Autodesk Inventor part; units mm, degrees
(part 4 of 4)
extrude "Extrusion2" cut sketch "Sketch2" against normal blind 1.5875 contours A0 L8 A2 L7 A1 L6 | L9 A4 L10 A5 L11 A3 | L12 A7 L14 A6 L13 A8 | L15 A11 L17 A10 L16 A9 | L18 A13 L20 A12 L19 A14 | L21 A17 L23 A16 L22 A15 | L24 A19 L26 A18 L25 A20 | L27 A23 L29 A22 L28 A21 | L30 A25 L32 A24 L31 A26 | L33 A29 L35 A28 L34 A27 | L36 A31 L38 A30 L37 A32 | L39 A35 L41 A34 L40 A33 | L42 A37 L44 A36 L43 A38 | L45 A41 L47 A40 L46 A39 | L48 A43 L50 A42 L49 A44 | L51 A47 L53 A46 L52 A45 | L54 A49 L56 A48 L55 A50 | L57 A53 L59 A52 L58 A51 | L60 A55 L62 A54 L61 A56 | L63 A59 L65 A58 L64 A57 | L66 A61 L68 A60 L67 A62 | L69 A65 L71 A64 L70 A63 | L72 A67 L74 A66 L73 A68 | L75 A71 L77 A70 L76 A69 | L78 A73 L80 A72 L79 A74 | L81 A77 L83 A76 L82 A75 | L84 A79 L86 A78 L85 A80 | L87 A83 L89 A82 L88 A81 | L90 A85 L92 A84 L91 A86 | L93 A89 L95 A88 L94 A87 | L96 A91 L98 A90 L97 A92 | L99 A95 L101 A94 L100 A93 | L102 A97 L104 A96 L103 A98 | L105 A101 L107 A100 L106 A99 | L108 A103 L110 A102 L109 A104 | L111 A107 L113 A106 L112 A105 | L114 A109 L116 A108 L115 A110 | L117 A113 L119 A112 L118 A111 | L120 A115 L122 A114 L121 A116 | L123 A119 L125 A118 L124 A117 | L126 A121 L128 A120 L127 A122 | L129 A125 L131 A124 L130 A123 | L132 A127 L134 A126 L133 A128 | L135 A131 L137 A130 L136 A129 | L138 A133 L140 A132 L139 A134 | L141 A137 L143 A136 L142 A135 | L144 A139 L146 A138 L145 A140 | L147 A143 L149 A142 L148 A141 | L150 A145 L152 A144 L151 A146 | L153 A149 L155 A148 L154 A147 | L156 A151 L158 A150 L157 A152 | L159 A155 L161 A154 L160 A153 | L162 A157 L164 A156 L163 A158 | L165 A161 L167 A160 L166 A159 | L168 A163 L170 A162 L169 A164 | L171 A167 L173 A166 L172 A165 | L174 A169 L176 A168 L175 A170 | L177 A173 L179 A172 L178 A171 | L180 A175 L182 A174 L181 A176 | L183 A179 L185 A178 L184 A177 | L186 A181 L188 A180 L187 A182 | L189 A185 L191 A184 L190 A183 | L192 A187 L194 A186 L193 A188 | L195 A191 L197 A190 L196 A189 | L198 A193 L200 A192 L199 A194 | L201 A197 L203 A196 L202 A195 | L204 A199 L206 A198 L205 A200 | L207 A203 L209 A202 L208 A201 | L210 A205 L212 A204 L211 A206 | L213 A209 L215 A208 L214 A207 | L216 A211 L218 A210 L217 A212 | L219 A215 L221 A214 L220 A213 | L222 A217 L224 A216 L223 A218 | L225 A221 L227 A220 L226 A219 | L228 A223 L230 A222 L229 A224 | L231 A227 L233 A226 L232 A225 | L234 A229 L236 A228 L235 A230 | L237 A233 L239 A232 L238 A231 | L240 A235 L242 A234 L241 A236 | L243 A239 L245 A238 L244 A237 | L246 A241 L248 A240 L247 A242 | L249 A245 L251 A244 L250 A243 | L252 A247 L254 A246 L253 A248 | L255 A251 L257 A250 L256 A249 | L258 A253 L260 A252 L259 A254 | L261 A257 L263 A256 L262 A255 | L264 A259 L266 A258 L265 A260 | L267 A263 L269 A262 L268 A261 | L270 A265 L272 A264 L271 A266 | L273 A269 L275 A268 L274 A267 | L276 A271 L278 A270 L277 A272 | L279 A275 L281 A274 L280 A273 | L282 A277 L284 A276 L283 A278 | L285 A281 L287 A280 L286 A279 | L288 A283 L290 A282 L289 A284 | L291 A287 L293 A286 L292 A285 | L294 A289 L296 A288 L295 A290 | L297 A293 L299 A292 L298 A291 | L300 A295 L302 A294 L301 A296 | L303 A299 L305 A298 L304 A297 | L306 A301 L308 A300 L307 A302 | L309 A305 L311 A304 L310 A303 | L312 A307 L314 A306 L313 A308 | L315 A311 L317 A310 L316 A309 | L318 A313 L320 A312 L319 A314 | L321 A317 L323 A316 L322 A315 | L324 A319 L326 A318 L325 A320 | L327 A323 L329 A322 L328 A321 | L330 A325 L332 A324 L331 A326 | L333 A329 L335 A328 L334 A327 | L336 A331 L338 A330 L337 A332 | L339 A335 L341 A334 L340 A333 | L342 A337 L344 A336 L343 A338 | L345 A341 L347 A340 L346 A339 | L348 A343 L350 A342 L349 A344 | L351 A347 L353 A346 L352 A345 | L354 A349 L356 A348 L355 A350 | L357 A353 L359 A352 L358 A351 | L360 A355 L362 A354 L361 A356 | L363 A359 L365 A358 L364 A357 | L366 A361 L368 A360 L367 A362 | L369 A365 L371 A364 L370 A363 | L372 A367 L374 A366 L373 A368 | L375 A371 L377 A370 L376 A369 | L378 A373 L380 A372 L379 A374 | L381 A377 L383 A376 L382 A375 | L384 A379 L386 A378 L385 A380 | L387 A383 L389 A382 L388 A381 | L390 A385 L392 A384 L391 A386 | L393 A389 L395 A388 L394 A387 | L396 A391 L398 A390 L397 A392 | L399 A395 L401 A394 L400 A393 | L402 A397 L404 A396 L403 A398 | L405 A401 L407 A400 L406 A399 | L408 A403 L410 A402 L409 A404 | L411 A407 L413 A406 L412 A405 | L414 A409 L416 A408 L415 A410 | L417 A413 L419 A412 L418 A411 | L420 A415 L422 A414 L421 A416 | L423 A419 L425 A418 L424 A417 | L426 A421 L428 A420 L427 A422 | L429 A425 L431 A424 L430 A423 | L432 A427 L434 A426 L433 A428 | L435 A431 L437 A430 L436 A429 | L438 A433 L440 A432 L439 A434 | L441 A437 L443 A436 L442 A435 | L444 A439 L446 A438 L445 A440 | L447 A443 L449 A442 L448 A441 | L450 A445 L452 A444 L451 A446 | L453 A449 L455 A448 L454 A447 | L456 A451 L458 A450 L457 A452 | L459 A455 L461 A454 L460 A453 | L462 A457 L464 A456 L463 A458 | L465 A461 L467 A460 L466 A459 | L468 A463 L470 A462 L469 A464 | L471 A467 L473 A466 L472 A465 | L474 A469 L476 A468 L475 A470 | L477 A473 L479 A472 L478 A471 | L480 A475 L482 A474 L481 A476 | L483 A479 L485 A478 L484 A477 | L486 A481 L488 A480 L487 A482 | L489 A485 L491 A484 L490 A483 | L492 A487 L494 A486 L493 A488 | L495 A491 L497 A490 L496 A489 | L498 A493 L500 A492 L499 A494 | L501 A497 L503 A496 L502 A495 | L504 A499 L506 A498 L505 A500 | L507 A503 L509 A502 L508 A501 | L510 A505 L512 A504 L511 A506 | L513 A509 L515 A508 L514 A507 | L516 A511 L518 A510 L517 A512 | L519 A515 L521 A514 L520 A513 | L522 A517 L524 A516 L523 A518 | L525 A521 L527 A520 L526 A519 | L528 A523 L530 A522 L529 A524 | L531 A527 L533 A526 L532 A525 | L534 A529 L536 A528 L535 A530 | L537 A533 L539 A532 L538 A531 | L540 A535 L542 A534 L541 A536 | L543 A539 L545 A538 L544 A537 | L546 A541 L548 A540 L547 A542 | L549 A545 L551 A544 L550 A543 | L552 A547 L554 A546 L553 A548 | L555 A551 L557 A550 L556 A549 | L558 A553 L560 A552 L559 A554 | L561 A557 L563 A556 L562 A555 | L564 A559 L566 A558 L565 A560 | L567 A563 L569 A562 L568 A561 | L570 A565 L572 A564 L571 A566 | L573 A569 L575 A568 L574 A567 | L576 A571 L578 A570 L577 A572 | L579 A575 L581 A574 L580 A573 | L582 A577 L584 A576 L583 A578 | L585 A581 L587 A580 L586 A579 | L588 A583 L590 A582 L589 A584 | L591 A587 L593 A586 L592 A585 | L594 A589 L596 A588 L595 A590 | L597 A593 L599 A592 L598 A591 | L600 A595 L602 A594 L601 A596 | L603 A599 L605 A598 L604 A597 | L606 A601 L608 A600 L607 A602 | L609 A605 L611 A604 L610 A603 | L612 A607 L614 A606 L613 A608 | L615 A611 L617 A610 L616 A609 | L618 A613 L620 A612 L619 A614 | L621 A617 L623 A616 L622 A615 | L624 A619 L626 A618 L625 A620 | L627 A623 L629 A622 L628 A621 | L630 A625 L632 A624 L631 A626 | L633 A629 L635 A628 L634 A627 | L636 A631 L638 A630 L637 A632 | L639 A635 L641 A634 L640 A633 | L642 A637 L644 A636 L643 A638 | L645 A641 L647 A640 L646 A639 | L648 A643 L650 A642 L649 A644 | L651 A647 L653 A646 L652 A645 | L654 A649 L656 A648 L655 A650 | L657 A653 L659 A652 L658 A651 | L660 A655 L662 A654 L661 A656 | L663 A659 L665 A658 L664 A657 | L666 A661 L668 A660 L667 A662 | L669 A665 L671 A664 L670 A663 | L672 A667 L674 A666 L673 A668 | L675 A671 L677 A670 L676 A669 | L678 A673 L680 A672 L679 A674 | L681 A677 L683 A676 L682 A675 | L684 A679 L686 A678 L685 A680 | L687 A683 L689 A682 L688 A681 | L690 A685 L692 A684 L691 A686 | L693 A689 L695 A688 L694 A687 | L696 A691 L698 A690 L697 A692 | L699 A695 L701 A694 L700 A693 | L702 A697 L704 A696 L703 A698 | L705 A701 L707 A700 L706 A699 | L708 A703 L710 A702 L709 A704 | L711 A707 L713 A706 L712 A705 | L714 A709 L716 A708 L715 A710 | L717 A713 L719 A712 L718 A711 | L720 A715 L722 A714 L721 A716 | L723 A719 L725 A718 L724 A717 | L726 A721 L728 A720 L727 A722 | L729 A725 L731 A724 L730 A723 | L732 A727 L734 A726 L733 A728 | L735 A731 L737 A730 L736 A729 | L738 A733 L740 A732 L739 A734 | L741 A737 L743 A736 L742 A735 | L744 A739 L746 A738 L745 A740 | L747 A743 L749 A742 L748 A741 | L750 A745 L752 A744 L751 A746 | L753 A749 L755 A748 L754 A747 | L756 A751 L758 A750 L757 A752 | L759 A755 L761 A754 L760 A753 | L762 A757 L764 A756 L763 A758 | L765 A761 L767 A760 L766 A759 | L768 A763 L770 A762 L769 A764 | L771 A767 L773 A766 L772 A765 | L774 A769 L776 A768 L775 A770 | L777 A773 L779 A772 L778 A771 | L780 A775 L782 A774 L781 A776 | L783 A779 L785 A778 L784 A777 | L786 A781 L788 A780 L787 A782 | L789 A785 L791 A784 L790 A783 | L792 A787 L794 A786 L793 A788 | L795 A791 L797 A790 L796 A789 | L798 A793 L800 A792 L799 A794 | L801 A797 L803 A796 L802 A795 | L804 A799 L806 A798 L805 A800 | L807 A803 L809 A802 L808 A801 | L810 A805 L812 A804 L811 A806 | L813 A809 L815 A808 L814 A807 | L816 A811 L818 A810 L817 A812 | L819 A815 L821 A814 L820 A813 | L822 A817 L824 A816 L823 A818 | L825 A821 L827 A820 L826 A819 | L828 A823 L830 A822 L829 A824 | L831 A827 L833 A826 L832 A825 | L834 A829 L836 A828 L835 A830 | L837 A833 L839 A832 L838 A831 | L840 A835 L842 A834 L841 A836 | L843 A839 L845 A838 L844 A837 | L846 A841 L848 A840 L847 A842 | L849 A845 L851 A844 L850 A843 | L852 A847 L854 A846 L853 A848 | L855 A851 L857 A850 L856 A849 | L858 A853 L860 A852 L859 A854 | L861 A857 L863 A856 L862 A855 | L864 A859 L866 A858 L865 A860 | L867 A863 L869 A862 L868 A861 | L870 A865 L872 A864 L871 A866 | L873 A869 L875 A868 L874 A867 | L876 A871 L878 A870 L877 A872 | L879 A875 L881 A874 L880 A873 | L882 A877 L884 A876 L883 A878 | L885 A881 L887 A880 L886 A879 | L888 A883 L890 A882 L889 A884 | L891 A887 L893 A886 L892 A885 | L894 A889 L896 A888 L895 A890 | L897 A893 L899 A892 L898 A891 | L900 A895 L902 A894 L901 A896 | L903 A899 L905 A898 L904 A897 | L906 A901 L908 A900 L907 A902 | L909 A905 L911 A904 L910 A903 | L912 A907 L914 A906 L913 A908 | L915 A911 L917 A910 L916 A909 | L918 A913 L920 A912 L919 A914 | L921 A917 L923 A916 L922 A915 | L924 A919 L926 A918 L925 A920 | L927 A923 L929 A922 L928 A921
body "Solid1"
